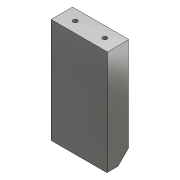
# Autodesk Inventor part: BC-10007
Saved by Autodesk Inventor 2016 (Build 200138000, 138)
## iProperties
Created: 2015-11-25
Part Number: BC-10007
Material: Aço Carbono AISI 1006
Document SubType Name: Modeling
Designer: reinaldo.basilio
Density: 7.87 g/cm^3
Appearance: Silver
Mass: 6238.06 g
Surface Area: 659.372 cm^2
Volume: 792.638 cm^3
Project: DIPOLO BC-3T- SIRIUS
Cost Center: 1504002005
Description: Peça frontal para fechar circuito  magnético.
Author: reinaldo.basilio
Subject: BC-10007
Title: DIPOLO BC-3T- SIRIUS
Autodesk Inventor part; units mm, degrees
ref_plane "YZ Plane" through (0, 0, 0) normal (1, 0, 0) x (0, 1, 0)
ref_plane "XZ Plane" through (0, 0, 0) normal (0, 1, 0) x (-1, 0, 0)
ref_plane "XY Plane" through (0, 0, 0) normal (0, 0, 1) x (1, 0, 0)
sketch "Sketch1" plane through (0, 0, 0) normal (0, 1, 0) x (-1, 0, 0)
  line L0 (52.5, 97.5) -> (-52.5, 97.5)
  line L1 (-52.5, 97.5) -> (-52.5, -97.5)
  line L2 (-52.5, -97.5) -> (52.5, -97.5)
  line L3 (52.5, -97.5) -> (52.5, 97.5)
  point P0 (0, 0)
  point P1 (0, -97.5)
  point P2 (-52.5, 0)
  dimension "d0" = 105
  dimension "d1" = 195
  constraints: 8 end point, 2 midpoint, 2 parallel, 1 horizontal, 1 horizontal alignment, 1 perpendicular, 1 vertical alignment
  measures "d0" distance of L1.end L2.end
  measures "d1" distance of L2.end L0.start
extrude "Extrusion1" add sketch "Sketch1" along normal blind 40
sketch "Sketch2" plane through (-52.5, 0, 97.5) normal (0, 0, 1) x (1, 0, 0)
  line L0 (0, 40) -> (105, 40)
  circle A0 centre (80, 20) radius 5
  circle A1 centre (25, 20) radius 5
  line L1 (105, 0) -> (105, 40) projected
  line L2 (0, 0) -> (105, 0) projected
  line L3 (52.5, 0) -> (52.5, -9.2371) construction
  point P0 (105, 20)
  dimension "d6" = 55
  dimension "d19" = 10
  dimension "d44" = 27.5
  constraints: 4 end point, 2 centre point, 2 horizontal alignment, 2 midpoint, 1 equal radius, 1 perpendicular
  measures "d6" distance of A1.centre A0.centre
  measures "d19" diameter of A0
  measures "d44" distance from line of L3 A0.centre
hole "Hole1" at (27.5, 20, 97.5) at (-27.5, 20, 97.5) direction (0, 0, -1) diameter 8.376 depth 20 tip angle 118 thread size "M10x1.5" class "6H" standard "ANSI Metric M Profile"
chamfer "Chamfer1" distance 20 angle 45 1 edges at (0, 40, -97.5)
sketch "Sketch3" plane through (52.5, 0, -97.5) normal (0, 0, -1) x (-1, 0, 0)
  line L0 (0, 20) -> (105, 20) projected
  line L1 (0, 0) -> (105, 0) projected
  circle A0 centre (25, 10) radius 4
  circle A1 centre (80, 10) radius 4
  point P0 (52.5, 0)
  dimension "d20" = 55
  dimension "d21" = 27.5
  dimension "d22" = 20
  dimension "d23" = 10
  dimension "d24" = 8
  constraints: 2 centre point, 1 equal radius, 1 horizontal alignment
  measures "d20" distance of A1.centre A0.centre
  measures "d21" horizontal distance of A0.centre point (52.5, 0)
  measures "d22" distance between parallel lines of L0 L1
  measures "d23" distance from line of A1.centre L1
  measures "d24" diameter of A0
hole "Hole2" at (27.5, 10, -97.5) at (-27.5, 10, -97.5) direction (0, 0, 1) diameter 4.917 depth 17.1 tip angle 118 thread size "M6x1" class "6H" standard "ISO Metric profile"
sketch "Sketch4" plane through (0, 40, 0) normal (0, 1, 0) x (1, 0, 0)
  circle A0 centre (-27.5, 40) radius 4
  circle A1 centre (27.5, 40) radius 4
  circle A2 centre (-27.5, -40) radius 4
  circle A3 centre (27.5, -40) radius 4
  line L0 (-52.5, -97.5) -> (52.5, -97.5) projected
  point P0 (0, 0)
  dimension "d32" = 8
  dimension "d33" = 55
  dimension "d34" = 27.5
  dimension "d35" = 80
  dimension "d46" = 57.5
  constraints: 4 centre point, 3 equal radius, 2 horizontal alignment, 2 vertical alignment
  measures "d32" diameter of A0
  measures "d33" distance of A1.centre A0.centre
  measures "d34" horizontal distance of point (0, 0) A0.centre
  measures "d35" distance of A2.centre A0.centre
  measures "d46" distance from line of L0 A2.centre
hole "Hole3" at (-27.5, 40, -40) at (27.5, 40, 40) at (-27.5, 40, 40) at (27.5, 40, -40) direction (0, -1, 0) diameter 6.647 depth 15 tip angle 118 thread size "M8x1.25" class "6H" standard "ISO Metric profile"
chamfer "Chamfer2" distance 1 angle 45 6 edges at (52.5, 40, 10) (-52.5, 40, 10) (-52.5, 30, -87.5) (52.5, 30, -87.5) (52.5, 10, -97.5) (-52.5, 10, -97.5)
equation "\"d44\" = 0.5 * d6"
equation "\"d21\" = 0.5 * d20"
equation "\"d23\" = 0.5 * d22"
equation "\"d34\" = 0.5 * d33"
body "Solid1"
